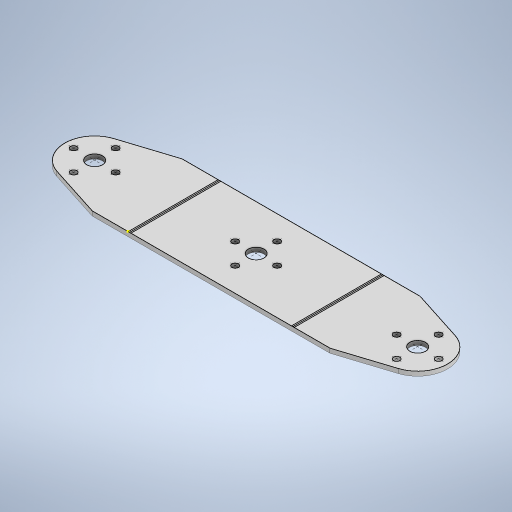
# Autodesk Inventor part: axis_5_bottom_frame
Saved by Autodesk Inventor 2024.2 (Build 282272000, 272)
## iProperties
Created: 2023-12-26
Part Number: axis_5_bottom_frame
Material: Generic
Document SubType Name: Modeling
Designer: chanh
Density: 1 g/cm^3
Appearance: Default
Author: chanh
Autodesk Inventor part; units mm, degrees
ref_plane "YZ Plane" through (0, 0, 0) normal (1, 0, 0) x (0, 1, 0)
ref_plane "XZ Plane" through (0, 0, 0) normal (0, 1, 0) x (-1, 0, 0)
ref_plane "XY Plane" through (0, 0, 0) normal (0, 0, 1) x (1, 0, 0)
sketch "Sketch1" plane through (0, 0, 0) normal (0, 1, 0) x (-1, 0, 0)
  line L0 (-54.9089, 0) -> (-54.9089, -30)
  line L1 (-0.4496, -30) -> (-0.4496, 0)
  circle A0 centre (-81.5486, -8) radius 1.05
  circle A1 centre (26.19, -8) radius 1.05
  circle A2 centre (-81.5486, -22) radius 1.05
  circle A3 centre (26.19, -22) radius 1.05
  circle A4 centre (-88.5486, -15) radius 1.05
  circle A5 centre (33.19, -15) radius 1.05
  circle A6 centre (-74.5486, -15) radius 1.05
  circle A7 centre (19.19, -15) radius 1.05
  circle A8 centre (-81.5486, -15) radius 2.6
  circle A9 centre (26.19, -15) radius 2.6
  circle A10 centre (-27.6793, -15) radius 2.6
  circle A11 centre (-27.6793, -22) radius 1.05
  circle A12 centre (-20.6793, -15) radius 1.05
  circle A13 centre (-27.6793, -8) radius 1.05
  circle A14 centre (-34.6793, -15) radius 1.05
  line L2 (-84.585, -24.4859) -> (-67.3586, -30)
  line L3 (12, -30) -> (29.2264, -24.4859)
  arc A15 (-84.585, -5.5141) -> (-84.585, -24.4859) centre (-81.5486, -15) ccw
  arc A16 (29.2264, -24.4859) -> (29.2264, -5.5141) centre (26.19, -15) ccw
  line L4 (-67.3586, 0) -> (-84.585, -5.5141)
  line L5 (29.2264, -5.5141) -> (12, 0)
  line L6 (-67.3586, 0) -> (12, 0)
  line L7 (12, -30) -> (-67.3586, -30)
  line L8 (-55.3586, -30) -> (-55.3586, 0)
  line L9 (-54.4593, 0) -> (-54.4593, -30)
  line L10 (-0.8993, -30) -> (-0.8993, 0)
  line L11 (0, 0) -> (0, -30)
  point P0 (0, 0)
  constraints: 24 end point, 17 centre point, 12 point on line, 6 vertical, 4 point on circle, 2 horizontal, 57 other
extrude "Extrusion1" add sketch "Sketch1" against normal blind 1.5
body "Solid1"
